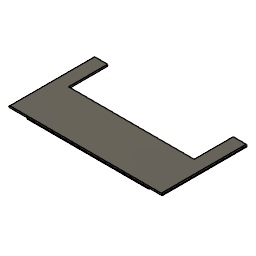
Ultra Half Frame Nikon F1-F6 (Autodesk Fusion 360 design; units mm, degrees)
Autodesk Fusion 360 part; units mm, degrees
note: some values were not read from the file. Set by a fixed rule: which sketch regions a step uses.
sketch "Sketch1" plane through (0, 0, 0) normal (0, 0, 1) x (1, 0, 0)
  line L0 (-25, 13) -> (11, 13)
  line L1 (-25, -0.2) -> (14.65, -0.2)
  line L2 (-25, -0.2) -> (-43.65, -0.2)
  line L3 (11, 24.2) -> (14.65, 24.2)
  line L4 (-43.65, 24.2) -> (-25, 24.2)
  line L5 (14.65, 24.2) -> (23.65, 24.2)
  line L6 (23.65, -0.2) -> (14.65, -0.2)
  line L7 (11, 13) -> (11, 24)
  line L8 (-25, 13) -> (-25, 24)
  line L9 (-43.65, -0.2) -> (-43.65, 24.2)
  line L10 (23.65, -0.2) -> (23.65, 24.2)
  line L11 (11, 24) -> (11, 24.2)
  line L12 (-25, 24) -> (-25, 24.2)
  constraint perpendicular L5 L7
  constraint perpendicular L4 L9
  constraint perpendicular L3 L11
  constraint perpendicular L4 L12
extrude "Extrude1" add sketch "Sketch1" along normal blind 0.48
sketch "Sketch10" plane through (0, 0, 0.48) normal (0, 0, 1) x (-1, 0, 0)
  line L0 (25, -13) -> (25, -24)
  line L1 (25, -24) -> (25, -24.2)
  line L2 (25, -24.2) -> (43.65, -24.2)
  line L3 (43.65, -24.2) -> (43.65, 0.2)
  line L4 (43.65, 0.2) -> (-23.65, 0.2)
  line L5 (-23.65, 0.2) -> (-23.65, -24.2)
  line L6 (-23.65, -24.2) -> (-11, -24.2)
  line L7 (-11, -24.2) -> (-11, -13)
  line L8 (-11, -13) -> (25, -13)
  line L9 (37.65, 0.2) -> (37.65, -24.2)
  dimension "d46" = 12.65
  constraint coincident L4 L9.start
  constraint coincident L2 L9.end
  constraint perpendicular L2 L9
  measures "d46" distance of L0 L9
extrude "Extrude13" cut sketch "Sketch10" against normal blind 2 contours L2 L3 L4 L9
sketch "Sketch11" plane through (0, 0, 0) normal (0, 0, -1) x (1, 0, 0)
  line L0 (-37.65, 0.2) -> (-37.65, -24.2)
  line L1 (-37.65, -24.2) -> (-25, -24.2)
  line L2 (-25, -24.2) -> (-25, -24)
  line L3 (-25, -24) -> (-25, -13)
  line L4 (-25, -13) -> (11, -13)
  line L5 (11, -13) -> (11, -24.2)
  line L6 (11, -24.2) -> (23.65, -24.2)
  line L7 (23.65, -24.2) -> (23.65, 0.2)
  line L8 (23.65, 0.2) -> (-37.65, 0.2)
  line L9 (10.5, -13) -> (10, -13)
  line L10 (10, -13) -> (10, -1)
  line L11 (10, -0.5) -> (10.5, -0.5)
  line L12 (10.5, -0.5) -> (10.5, -13)
  line L13 (-24.5, -13) -> (-24, -13)
  line L14 (-24, -13) -> (-24, -1)
  line L15 (-24, -0.5) -> (-24.5, -0.5)
  line L16 (-24.5, -0.5) -> (-24.5, -13)
  line L17 (-24.5, -0.5) -> (10.5, -0.5)
  line L18 (10.5, -0.5) -> (10.5, -1)
  line L19 (10, -1) -> (-24, -1)
  line L20 (-24.5, -1) -> (-24.5, -0.5)
  point P0 (11, -13)
  point P1 (10.75, -13)
  point P2 (-25, -13)
  point P3 (-24.75, -13)
  point P4 (11, 0)
  point P5 (11, -0.25)
  point P6 (10.75, -0.25)
  dimension "d49" = 0.25
  dimension "d50" = 0.25
  dimension "d51" = 0.25
  dimension "d52" = 0.25
  constraint coincident P0 L4.end
  constraint coincident L4 P1
  constraint coincident P2 L3.end
  constraint coincident L4 P3
  constraint horizontal L9
  constraint vertical L10
  constraint horizontal L11
  constraint vertical L12
  constraint coincident L4 L9.start
  constraint horizontal L13
  constraint vertical L14
  constraint horizontal L15
  constraint vertical L16
  constraint coincident L4 L13.start
  constraint horizontal L17
  constraint vertical L18
  constraint horizontal L19
  constraint vertical L20
  constraint coincident L12 L18.end
  measures "d49" distance of P0 P1
  measures "d50" distance of P2 P3
  measures "d51" distance of P4 P5
  measures "d52" distance of P5 P6
extrude "Extrude14" add sketch "Sketch11" along normal blind 1 contours L4 L9 L10 L11 L12 L13 L14 L15 L16 L17 L18 L19 L20
sketch "Sketch12" plane through (0, 0, 0.48) normal (0, 0, 1) x (-1, 0, 0)
  line L0 (37.65, -24.2) -> (37.65, 0.2)
  line L1 (37.65, 0.2) -> (-23.65, 0.2)
  line L2 (-23.65, 0.2) -> (-23.65, -24.2)
  line L3 (-23.65, -24.2) -> (-11, -24.2)
  line L4 (-11, -24.2) -> (-11, -13)
  line L5 (-11, -13) -> (25, -13)
  line L6 (25, -13) -> (25, -24)
  line L7 (25, -24) -> (25, -24.2)
  line L8 (25, -24.2) -> (37.65, -24.2)
  line L9 (-15, -24.2) -> (-15, 0.2) construction
  line L10 (29, 0.2) -> (29, -24.2) construction
  line L11 (-15, 0.2) -> (-15, -24.2) construction
  line L12 (-15, 0.2) -> (-15, -24.2)
  line L13 (29, -24.2) -> (29, 0.2)
  dimension "d57" = 4
  dimension "d58" = 4
  constraint coincident L3 L9.start
  constraint coincident L1 L9.end
  constraint perpendicular L1 L9
  constraint coincident L8 L10.end
  constraint perpendicular L8 L10
  measures "d57" distance of L4 L9
  measures "d58" distance of L6 L10
extrude "Extrude15" cut sketch "Sketch12" against normal blind 0.48 contours L0 L1 L8 L13 | L1 L2 L3 L12
fillet "Fillet2" radius 0.24 2 edges at (15, 12, 0.48) (-29, 12, 0.48)
equation "d9 = 0.12 mm * 4"
equation "d62 = ( 0.48 / 2 ) * 1 mm"
